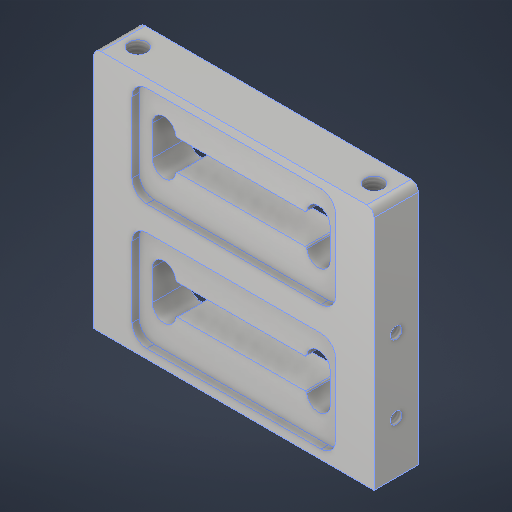
# Autodesk Inventor part: Spulenhalter Hinten
Saved by Autodesk Inventor 2025.2 (Build 292293000, 293)
## iProperties
Part Number: Spulenhalter Hinten
Material: Aluminium 6061
Document SubType Name: Modeling
Designer: rYan
Density: 2.7 g/cm^3
Appearance: Aluminium - flach
Mass: 16.9891 g
Surface Area: 44.1608 cm^2
Volume: 6.29226 cm^3
Author: rYan
Autodesk Inventor part; units mm, degrees
ref_plane "YZ Plane" through (0, 0, 0) normal (1, 0, 0) x (0, 1, 0)
ref_plane "XZ Plane" through (0, 0, 0) normal (0, 1, 0) x (-1, 0, 0)
ref_plane "XY Plane" through (0, 0, 0) normal (0, 0, 1) x (1, 0, 0)
sketch "Skizze1" plane through (0, 0, 0) normal (0, 1, 0) x (-1, 0, 0)
  line L0 (-19, 0) -> (-19, 30)
  line L1 (19, 30) -> (19, 0)
  line L2 (-12.05, 3) -> (-12.05, 7.1)
  line L3 (-8.85, 7.1) -> (8.85, 7.1)
  line L4 (12.05, 7.1) -> (12.05, 3)
  line L5 (8.85, 19.95) -> (-8.85, 19.95)
  line L6 (-12.05, 19.95) -> (-12.05, 24.05)
  line L7 (-8.85, 24.05) -> (8.85, 24.05)
  line L8 (12.05, 24.05) -> (12.05, 19.95)
  arc A0 (12.05, 24.05) -> (8.85, 24.05) centre (10.45, 24.05) ccw
  arc A1 (8.85, 19.95) -> (12.05, 19.95) centre (10.45, 19.95) ccw
  arc A2 (-8.85, 24.05) -> (-12.05, 24.05) centre (-10.45, 24.05) ccw
  arc A3 (-12.05, 19.95) -> (-8.85, 19.95) centre (-10.45, 19.95) ccw
  arc A4 (12.05, 7.1) -> (8.85, 7.1) centre (10.45, 7.1) ccw
  arc A5 (-8.85, 7.1) -> (-12.05, 7.1) centre (-10.45, 7.1) ccw
  line L9 (-8.85, 3) -> (8.85, 3)
  arc A6 (8.85, 3) -> (12.05, 3) centre (10.45, 3) ccw
  arc A7 (-12.05, 3) -> (-8.85, 3) centre (-10.45, 3) ccw
  line L10 (19, -3) -> (-19, -3)
  line L11 (-19, -3) -> (-19, 0)
  line L12 (19, 0) -> (19, -3)
  line L13 (0, 30) -> (19, 30)
  line L14 (19, 30) -> (-19, 30)
  arc A8 (-12.3, 19.95) -> (-8.617, 19.7) centre (-10.45, 19.95) ccw
  line L15 (-8.617, 19.7) -> (8.617, 19.7)
  arc A9 (8.617, 19.7) -> (12.3, 19.95) centre (10.45, 19.95) ccw
  line L16 (12.3, 19.95) -> (12.3, 24.05)
  arc A10 (12.3, 24.05) -> (8.617, 24.3) centre (10.45, 24.05) ccw
  line L17 (8.617, 24.3) -> (-8.617, 24.3)
  arc A11 (-8.617, 24.3) -> (-12.3, 24.05) centre (-10.45, 24.05) ccw
  line L18 (-12.3, 24.05) -> (-12.3, 19.95)
  line L19 (8.617, 7.35) -> (-8.617, 7.35)
  arc A12 (-8.617, 7.35) -> (-12.3, 7.1) centre (-10.45, 7.1) ccw
  line L20 (-12.3, 7.1) -> (-12.3, 3)
  arc A13 (-12.3, 3) -> (-8.617, 2.75) centre (-10.45, 3) ccw
  line L21 (-8.617, 2.75) -> (8.617, 2.75)
  arc A14 (8.617, 2.75) -> (12.3, 3) centre (10.45, 3) ccw
  line L22 (12.3, 3) -> (12.3, 7.1)
  arc A15 (12.3, 7.1) -> (8.617, 7.35) centre (10.45, 7.1) ccw
  point P0 (0, 22)
  point P1 (19, 0)
  dimension "d94" = 0.25
  dimension "d115" = 0.25
  constraints: 46 end point, 32 point on circle, 16 centre point, 8 parallel, 7 tangent, 5 point on line, 3 horizontal, 3 perpendicular, 2 collinear, 13 other
  measures "d94" distance between parallel lines of L7 L17
  measures "d115" distance between parallel lines of L3 L19
extrude "Grundkörper" add sketch "Skizze1" along normal mid plane 6 contours L0 L14 L13 L1 L12 L10 L11 | L18 A11 L17 A10 L16 A9 L15 A8 | A15 L22 A14 L21 A13 L20 A12 L19
sketch "Skizze2" plane through (0, -3, 0) normal (0, -1, 0) x (1, 0, 0)
  line L0 (-11.8, 15.2) -> (11.8, 15.2)
  line L1 (13.8, 17.2) -> (13.8, 26.8)
  line L2 (11.8, 28.8) -> (-11.8, 28.8)
  line L3 (-13.8, 26.8) -> (-13.8, 17.2)
  arc A0 (-11.8, 28.8) -> (-13.8, 26.8) centre (-11.8, 26.8) ccw
  arc A1 (-13.8, 17.2) -> (-11.8, 15.2) centre (-11.8, 17.2) ccw
  arc A2 (11.8, 15.2) -> (13.8, 17.2) centre (11.8, 17.2) ccw
  arc A3 (13.8, 26.8) -> (11.8, 28.8) centre (11.8, 26.8) ccw
  line L4 (19, 0) -> (-19, 0) projected
  line L5 (-19, 0) -> (19, 0) construction
  line L6 (-11.8, -1.75) -> (11.8, -1.75)
  line L7 (13.8, 0.25) -> (13.8, 9.85)
  line L8 (11.8, 11.85) -> (-11.8, 11.85)
  line L9 (-13.8, 9.85) -> (-13.8, 0.25)
  arc A4 (-11.8, 11.85) -> (-13.8, 9.85) centre (-11.8, 9.85) ccw
  arc A5 (-13.8, 0.25) -> (-11.8, -1.75) centre (-11.8, 0.25) ccw
  arc A6 (11.8, -1.75) -> (13.8, 0.25) centre (11.8, 0.25) ccw
  arc A7 (13.8, 9.85) -> (11.8, 11.85) centre (11.8, 9.85) ccw
  constraints: 16 end point, 16 point on circle, 16 tangent, 8 centre point, 6 equal radius, 4 parallel, 2 horizontal, 2 perpendicular
extrude "Tasche" cut sketch "Skizze2" against normal blind 1
sketch "Skizze10" plane through (19, 3, -3) normal (0, 0, -1) x (-1, 0, 0)
  line L0 (-3.4, -3) -> (41.4, -3)
  line L1 (19, 19.4) -> (19, -25.4)
  point P0 (19, -3)
  point P1 (19, -3)
  point P2 (3, -3)
  point P3 (35, -3)
  dimension "d96" = 32
  constraints: 4 end point, 2 point on line, 1 symmetric about line
  measures "d96" distance of point (35, -3) point (3, -3)
hole "Fixierung" at (16, 0, -3) at (-16, 0, -3) direction (0, 0, 1) diameter 3.242 depth 6 tip angle 118 thread size "M4x0.7" class "6H" standard "ISO Metric profile"
fillet "Rundung1" radius 1 2 edges at (-19, 0, 30) (19, 0, 30)
fillet "Rundung2" radius 0.2 8 edges at (-8.85, 0.5, 24.05) (8.85, 0.5, 24.05) (-8.85, 0.5, 19.95) (8.85, 0.5, 19.95) (-8.85, 0.5, 3) (8.85, 0.5, 3) (-8.85, 0.5, 7.1) (8.85, 0.5, 7.1)
sketch "Skizze11" plane through (19, -3, -3) normal (1, 0, 0) x (0, 0, -1)
  point P0 (-7, 3)
  point P1 (-17, 3)
hole "Federn" at (19, 0, 4) at (19, 0, 14) direction (-1, 0, 0) diameter 1.567 depth 4 tip angle 118 thread size "M2x0.4" class "6H" standard "ISO Metric profile"
mirror "Spiegeln1" about plane through (0, 0, 0) normal (1, 0, 0) of "Federn"
sketch "Skizze12" plane through (-18, 3, 30) normal (0, 0, 1) x (1, 0, 0)
  line L0 (18, -3) -> (2, -3)
  line L1 (18, -3) -> (18, 0)
  line L2 (26.6611, 0) -> (9.3389, 0) projected
  point P0 (34, -3)
  dimension "d117" = 16
  constraints: 4 end point, 1 coincident, 1 horizontal, 1 midpoint, 1 symmetric about line
  measures "d117" distance of L0.start L0.end
hole "Platinenhalterung" at (-16, 0, 30) at (16, 0, 30) direction (0, 0, -1) diameter 2.459 depth 6 tip angle 118 thread size "M3x0.5" class "6H" standard "ISO Metric profile"
